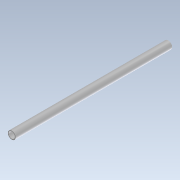
# Autodesk Inventor part: Upper_Arm_Shaft
Saved by Autodesk Inventor 2021.4 (Build 254397000, 397)
## iProperties
Created: 2022-07-05
Part Number: Upper_Arm_Shaft
Material: Aluminum 6061
Document SubType Name: Modeling
Designer: alexw
Mass: 15.2681 g
Surface Area: 113.663 cm^2
Volume: 5.65487 cm^3
Density: 2.7 g/cm^3
Appearance: Aluminum - Flat
Shaft_DiaOut: 10,000 mm
Shaft_DiaIn: 8,000 mm
Author: alexw
Autodesk Inventor part; units mm, degrees
ref_plane "YZ Plane" through (0, 0, 0) normal (1, 0, 0) x (0, 1, 0)
ref_plane "XZ Plane" through (0, 0, 0) normal (0, 1, 0) x (-1, 0, 0)
ref_plane "XY Plane" through (0, 0, 0) normal (0, 0, 1) x (1, 0, 0)
sketch "Sketch1" plane through (0, 0, 0) normal (0, 0, 1) x (1, 0, 0)
  circle A0 centre (0, 0) radius 5
  circle A1 centre (0, 0) radius 4
  dimension "Shaft_DiaOut" = 10
  dimension "Shaft_DiaIn" = 8
  constraints: 2 centre point, 2 coincident
  measures "Shaft_DiaOut" diameter of A0
  measures "Shaft_DiaIn" diameter of A1
extrude "Extrusion1" add sketch "Sketch1" along normal blind 200
body "Solid1"
